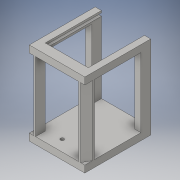
# Autodesk Inventor part: Body
Saved by Autodesk Inventor 2016 (Build 200138000, 138)
## iProperties
Created: 2018-10-20
Part Number: Body
Material: Generic
Document SubType Name: Modeling
Designer: Kyle
Density: 1 g/cm^3
Appearance: Default
Author: Kyle
Autodesk Inventor part; units mm, degrees
ref_plane "YZ Plane" through (0, 0, 0) normal (1, 0, 0) x (0, 1, 0)
ref_plane "XZ Plane" through (0, 0, 0) normal (0, 1, 0) x (-1, 0, 0)
ref_plane "XY Plane" through (0, 0, 0) normal (0, 0, 1) x (1, 0, 0)
sketch "Sketch1" plane through (0, 0, 0) normal (0, 1, 0) x (-1, 0, 0)
  line L0 (-40, -47.5) -> (40, -47.5)
  line L1 (40, -47.5) -> (40, 47.5)
  line L2 (40, 47.5) -> (-40, 47.5)
  line L3 (-40, 47.5) -> (-40, -47.5)
  line L4 (-40, -47.5) -> (40, 47.5) construction
  line L5 (40, -47.5) -> (-40, 47.5) construction
  line L6 (0, 0) -> (0, -31.5)
  line L7 (0, -31.5) -> (8.5, -31.5)
  line L8 (0, 0) -> (2.25, 0)
  line L9 (0, 0) -> (0, 17.5)
  line L10 (0, 17.5) -> (0, 19)
  line L11 (0, 19) -> (24, 19)
  line L12 (0, -17.5) -> (0, -19)
  line L13 (0, 31.5) -> (-19.5, 31.5)
  line L14 (0, 0) -> (0, 31.5)
  line L15 (0, 31.5) -> (8.5, 31.5)
  circle A0 centre (8.5, 31.5) radius 2.5
  line L16 (0, -19) -> (24, -19)
  circle A1 centre (24, -19) radius 2.5
  line L17 (0, 0) -> (0, -17.5)
  circle A2 centre (-19.5, 31.5) radius 2.5
  circle A3 centre (-19.5, 31.5) radius 2.5
  point P0 (0.5, 0.75)
  point P1 (0.5, -0.75)
  dimension "d0" = 80
  dimension "d1" = 95
  dimension "d2" = 17.5
  dimension "d3" = 8.5
  dimension "d5" = 31.5
  dimension "d6" = 24
  dimension "d7" = 2.25
  dimension "d12" = 19.5
  constraints: 36 end point, 6 symmetric about line, 4 centre point, 4 horizontal, 4 point on line, 3 perpendicular, 2 midpoint, 2 parallel, 2 vertical, 1 coincident, 1 other
  measures "d0" distance of L3.start L1.end
  measures "d1" distance of L1.start L1.end
  measures "d2" distance of L6.start L10.start
  measures "d3" distance of L7.start L7.end
  measures "d5" distance of L6.start L7.start
  measures "d6" distance of L11.start L11.end
  measures "d7" distance of L8.start L8.end
  measures "d12" distance of L15.start L13.end
extrude "Extrusion1" add sketch "Sketch1" along normal blind 10
sketch "Sketch2" plane through (0, 10, 0) normal (0, 1, 0) x (1, 0, 0)
  line L0 (-40, -47.5) -> (40, -47.5) projected
  line L1 (-40, -47.5) -> (-40, -36.5)
  line L2 (-40, 47.5) -> (-40, -47.5) projected
  line L3 (-40, -36.5) -> (-33.6491, -47.5)
  line L4 (-40, -36.5) -> (-27.2983, -36.5) construction
  line L5 (-33.6491, -47.5) -> (-33.6491, -43.5)
  line L6 (-40, -36.5) -> (-40, -33.5)
  line L7 (-33.6491, -47.5) -> (-33.6491, -45.5)
  line L8 (-32.6491, -47.5) -> (-31.6491, -47.5)
  line L9 (0, 0) -> (0, -47.5)
  line L10 (-40, -33.5) -> (-31, -33.5)
  line L11 (-31, -33.5) -> (-31, -47.5)
  line L12 (-33.6491, -47.5) -> (-31, -47.5)
  line L13 (40, -47.5) -> (40, -36.5)
  line L14 (40, -36.5) -> (33.6491, -47.5)
  line L15 (40, -36.5) -> (27.2983, -36.5) construction
  line L16 (33.6491, -47.5) -> (33.6491, -43.5)
  line L17 (40, -36.5) -> (40, -33.5)
  line L18 (33.6491, -47.5) -> (33.6491, -45.5)
  line L19 (32.6491, -47.5) -> (31.6491, -47.5)
  line L20 (40, -33.5) -> (31, -33.5)
  line L21 (31, -33.5) -> (31, -47.5)
  line L22 (33.6491, -47.5) -> (31, -47.5)
  line L23 (-40, 47.5) -> (-31, 47.5)
  line L24 (-31, 47.5) -> (-31, 33.5)
  line L25 (-31, 33.5) -> (-40, 33.5)
  line L26 (-40, 33.5) -> (-40, 47.5)
  line L27 (40, -47.5) -> (40, 47.5) projected
  line L28 (40, 47.5) -> (31, 47.5)
  line L29 (31, 47.5) -> (31, 33.5)
  line L30 (31, 33.5) -> (40, 33.5)
  line L31 (40, 33.5) -> (40, 47.5)
  dimension "d15" = 11
  dimension "d16" = 60
  dimension "d18" = 3
  dimension "d20" = 2
  dimension "d21" = 9
  dimension "d22" = 9
  dimension "d23" = 14
  dimension "d24" = 9
  dimension "d25" = 14
  constraints: 58 end point, 10 symmetric about line, 6 point on line, 4 horizontal, 4 parallel, 4 perpendicular, 3 midpoint, 1 collinear, 1 equal length
  measures "d15" distance of L0.start L1.end
  measures "d16" angle of L3 L4
  measures "d18" distance of L1.end L6.end
  measures "d20" distance of L3.end L7.end
  measures "d21" distance of L6.end L10.end
  measures "d22" distance of L24.end L25.end
  measures "d23" distance of L23.end L24.end
  measures "d24" distance of L30.end L29.end
  measures "d25" distance of L28.end L29.end
extrude "Extrusion2" add sketch "Sketch2" along normal blind 100 contours L2 L23 L24 L25 | L30 L29 L28 L27 | L21 L20 L17 L14 L0 | L3 L2 L10 L11 L0
sketch "Sketch4" plane through (0, 110, 0) normal (0, 1, 0) x (1, 0, 0)
  line L0 (-40, 47.5) -> (-40, 33.5) projected
  line L1 (-40, 33.5) -> (-31, 33.5) projected
  line L2 (-31, 33.5) -> (-31, 47.5) projected
  line L3 (-31, 47.5) -> (-40, 47.5) projected
  line L4 (40, 47.5) -> (31, 47.5) projected
  line L5 (31, 47.5) -> (31, 33.5) projected
  line L6 (31, 33.5) -> (40, 33.5) projected
  line L7 (40, 33.5) -> (40, 47.5) projected
  line L8 (33.6491, -47.5) -> (40, -36.5) projected
  line L9 (40, -36.5) -> (40, -33.5) projected
  line L10 (40, -33.5) -> (31, -33.5) projected
  line L11 (31, -33.5) -> (31, -47.5) projected
  line L12 (31, -47.5) -> (33.6491, -47.5) projected
  line L13 (-31, -47.5) -> (-31, -33.5) projected
  line L14 (-33.6491, -47.5) -> (-31, -47.5) projected
  line L15 (-31, -47.5) -> (-31, -33.5) projected
  line L16 (-31, -33.5) -> (-40, -33.5) projected
  line L17 (-40, -33.5) -> (-40, -36.5) projected
  line L18 (-40, -36.5) -> (-33.6491, -47.5) projected
  line L19 (-33.6491, -47.5) -> (-40, -36.5) projected
  line L20 (-40, -36.5) -> (-40, -47.5) projected
  line L21 (-40, -47.5) -> (-33.6491, -47.5) projected
  line L22 (40, -36.5) -> (33.6491, -47.5) projected
  line L23 (33.6491, -47.5) -> (40, -47.5) projected
  line L24 (40, -47.5) -> (40, -36.5) projected
  line L25 (-40, 47.5) -> (40, 47.5) projected
  line L26 (-40, 47.5) -> (-40, -47.5)
  line L27 (40, -47.5) -> (-40, -47.5) projected
  line L28 (-40, -47.5) -> (40, -47.5)
  line L29 (40, -47.5) -> (40, 47.5)
  line L30 (31, 33.5) -> (31, 47.5) projected
  line L31 (31, 47.5) -> (40, 47.5)
  line L32 (31, 47.5) -> (31, -33.5)
  line L33 (40, -33.5) -> (31, -33.5) projected
  line L34 (-40, -33.5) -> (-31, -33.5) projected
  line L35 (31, -33.5) -> (-31, -33.5)
  line L36 (-31, -33.5) -> (-31, 47.5)
  line L37 (-31, 47.5) -> (-31, 33.5) projected
  line L38 (-40, 47.5) -> (-31, 47.5)
  line L39 (-31, 47.1909) -> (-31, 33.5)
  line L40 (-40, 47.5) -> (-40, 33.5) projected
  line L41 (-31, 33.5) -> (-40, 33.5)
  line L42 (31, 33.5) -> (40, 33.5) projected
  line L43 (31, 33.5) -> (40, 33.5)
  point P0 (0, 0)
  constraints: 22 end point, 6 perpendicular, 3 horizontal, 1 collinear, 1 point on line, 1 vertical, 1 other
extrude "Extrusion3" add sketch "Sketch4" along normal blind 10 contours L3 L2 L1 L0 | L1 L36 L16 L26 | L16 L13 L14 L18 L17 | L4 L7 L6 L5 | L35 L11 L27 L13 | L18 L21 L20 | L6 L29 L10 L32 | L10 L9 L8 L12 L11 | L8 L24 L23
sketch "Sketch5" plane through (40, 0, -47.5) normal (0, 0, -1) x (-1, 0, 0)
  line L0 (80, 0) -> (0, 0) projected
  line L1 (80, 0) -> (80, 120) projected
  line L2 (71, 120) -> (80, 120) projected
  line L3 (71, 10) -> (71, 120) projected
  line L4 (9, 10) -> (71, 10) projected
  line L5 (9, 10) -> (9, 120) projected
  line L6 (0, 120) -> (9, 120) projected
  line L7 (0, 0) -> (0, 120) projected
  line L8 (9, 110) -> (71, 110) projected
  line L9 (71, 110) -> (71, 120) projected
  line L10 (9, 120) -> (71, 120) projected
  line L11 (9, 110) -> (9, 120) projected
  line L12 (9, 110) -> (9, 113)
  line L13 (9, 10) -> (9, 120) projected
  line L14 (9, 113) -> (4.5, 113)
  line L15 (4.5, 113) -> (4.5, 117)
  line L16 (4.5, 117) -> (9, 117)
  line L17 (9, 117) -> (9, 113)
  line L18 (9, 117) -> (9, 113)
  line L19 (9, 113) -> (71, 113)
  line L20 (71, 10) -> (71, 120) projected
  line L21 (71, 113) -> (75.5, 113)
  line L22 (75.5, 113) -> (75.5, 117)
  line L23 (75.5, 117) -> (71, 117)
  line L24 (71, 113) -> (71, 117)
  line L25 (71, 113) -> (71, 117)
  line L26 (8.545, 117) -> (71, 117)
  point P0 (40, 0)
  dimension "d30" = 3
  dimension "d31" = 4
  dimension "d32" = 4
  constraints: 26 end point, 6 perpendicular, 6 point on line, 4 collinear
  measures "d30" distance of L8.start L12.end
  measures "d31" distance of L14.end L15.end
  measures "d32" distance of L21.end L22.end
extrude "Extrusion4" cut sketch "Sketch5" against normal blind 88 contours L23 L22 L21 L3 | L3 L19 L5 L26 | L5 L14 L15 L16
sketch "Sketch6" plane through (0, 0, 0) normal (0, -1, 0) x (1, 0, 0)
  point P0 (0, 0)
body "Solid1"
